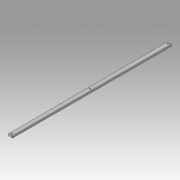
# Autodesk Inventor part: x-lift arm prototype piece
Saved by Autodesk Inventor 2016 (Build 200138000, 138)
## iProperties
Created: 2015-12-16
Part Number: x-lift arm prototype piece
Material: Generic
Document SubType Name: Modeling
Designer: Delta
Density: 1 g/cm^3
Appearance: Default
Author: Delta
Autodesk Inventor part; units mm, degrees
ref_plane "YZ Plane" through (0, 0, 0) normal (1, 0, 0) x (0, 1, 0)
ref_plane "XZ Plane" through (0, 0, 0) normal (0, 1, 0) x (-1, 0, 0)
ref_plane "XY Plane" through (0, 0, 0) normal (0, 0, 1) x (1, 0, 0)
sketch "Sketch1" plane through (0, 0, 0) normal (0, 0, 1) x (1, 0, 0)
  line L0 (0, 0) -> (12.7, 0)
  line L1 (12.7, 0) -> (12.7, 6.35)
  line L2 (12.7, 6.35) -> (0, 6.35)
  line L3 (0, 6.35) -> (0, 0)
  dimension "d0" = 12.7
  dimension "d1" = 6.35
  constraints: 8 end point, 2 parallel, 1 horizontal, 1 perpendicular
  measures "d0" distance of L2.end L1.end
  measures "d1" distance of L1.end L0.end
extrude "Extrusion1" add sketch "Sketch1" along normal blind 444.5
chamfer "Chamfer2" distance 1.27 angle 45 12 edges at (12.7, 0, 222.25) (0, 0, 222.25) (12.7, 6.35, 222.25) (0, 6.35, 222.25) (6.35, 0, 444.5) (6.35, 6.35, 444.5) (6.35, 0, 0) (6.35, 6.35, 0) (12.7, 3.175, 0) (0, 3.175, 0) (0, 3.175, 444.5) (12.7, 3.175, 444.5)
sketch "Sketch3" plane through (1.27, 6.35, 1.27) normal (0, 1, 0) x (1, 0, 0)
  line L0 (10.16, 0) -> (10.16, -441.96) projected
  line L1 (0, 0) -> (10.16, 0) projected
  line L2 (0, -441.96) -> (10.16, -441.96) projected
  point P0 (-1.27, 1.27)
  point P1 (5.08, -3.81)
  point P2 (5.08, -220.98)
  point P3 (5.08, -438.15)
  point P4 (22.86, 0)
  point P5 (22.86, -441.96)
  dimension "d17" = 5.08
  dimension "d18" = 3.81
  dimension "d19" = 5.08
  dimension "d20" = 3.81
  dimension "d21" = 5.08
  dimension "d22" = 220.98
  constraints: 1 other
  measures "d18" distance from line of L1 point (5.08, -3.81)
  measures "d20" distance from line of L2 point (5.08, -438.15)
  measures "d22" distance from line of L2 point (5.08, -220.98)
hole "Hole1" at (6.35, 6.35, 5.08) at (6.35, 6.35, 222.25) at (6.35, 6.35, 439.42) direction (0, -1, 0) diameter 3.81 end through all
equation "\"d19\" = d17"
equation "\"d20\" = d18"
equation "\"d21\" = d17"
body "Solid1"
